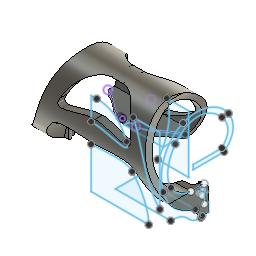
battery (Autodesk Fusion 360 design; units mm, degrees)
Autodesk Fusion 360 part; units mm, degrees
sketch "Skizze5" plane through (0, 0, 0) normal (0, 0, 1) x (1, 0, 0)
  line L0 (28.5, 22, 10) -> (28.5, 20, 10)
  line L1 (28.5, 20, 10) -> (29.5, 21, 10)
  line L2 (29.5, 21, 10) -> (29.5, 19, 10)
  line L3 (28.5, 22, 10) -> (31, 22, 10)
  line L4 (31, 22, 10) -> (31, 19, 10)
  line L5 (29.5, 19, 10) -> (31, 19, 10)
sketch "Skizze6" plane through (0, 0, 0) normal (1, 0, 0) x (0, 1, 0)
  line L0 (29, 22, 31) -> (15, 22, 31)
  line L1 (15, 22, 31) -> (15, 24, 31)
  spline S0 degree 5 poles (14, 14, 31) (13.4292, 14.0943, 31) (12.3218, 14.3255, 31) (10.7626, 14.7996, 31) (8.8887, 15.6876, 31) (6.9008, 17.2273, 31) (5.2976, 19.1966, 31) (4.1324, 21.5861, 31) (3.4909, 24.3735, 31) (3.4767, 27.5066, 31) (4.1857, 30.8831, 31) (5.682, 34.3253, 31) (7.9761, 37.5659, 31) (10.9879, 40.2008, 31) (14.6077, 41.7896, 31) (18.6539, 41.9776, 31) (22.843, 40.5947, 31) (26.7442, 37.7833, 31) (29.7595, 34.0835, 31) (31.0103, 30.6651, 31) (30.6995, 27.8746, 31) (29.6969, 26.1358, 31) (28.8446, 25.0136, 31) (28.2808, 24.3276, 31) (28, 24, 31) knots 0 0 0 0 0 0 0.05 0.1 0.15 0.2 0.25 0.3 0.35 0.4 0.45 0.5 0.55 0.6 0.65 0.7 0.75 0.8 0.85 0.9 0.95 1 1 1 1 1 1
  line L2 (23, 42, 31) -> (33, 30, 31)
  line L3 (31, 27.5, 31) -> (25, 20.5, 31)
  line L4 (15, 24, 31) -> (28, 24, 31)
  line L5 (3.1603, 30.7591, 31) -> (10.8397, 41.2409, 31)
  line L6 (14, 14, 31) -> (20, 14, 31)
  spline S1 degree 5 poles (16, 6.056, 31) (15.2365, 6.3099, 31) (13.7317, 6.851, 31) (11.5407, 7.7632, 31) (8.7707, 9.2347, 31) (5.6767, 11.7695, 31) (3.1232, 15.2227, 31) (1.3063, 19.671, 31) (0.4544, 24.7581, 31) (0.7322, 29.8853, 31) (2.1659, 34.6408, 31) (4.6898, 38.6535, 31) (8.1453, 41.6577, 31) (12.2989, 43.4702, 31) (16.8454, 44.0079, 31) (21.4291, 43.2885, 31) (25.6792, 41.4221, 31) (29.2431, 38.6264, 31) (31.8178, 35.1939, 31) (33.1909, 31.5811, 31) (33.2558, 28.0905, 31) (32.2282, 25.503, 31) (30.8496, 23.6989, 31) (29.6614, 22.5563, 31) (29, 22, 31) knots 0 0 0 0 0 0 0.05 0.1 0.15 0.2 0.25 0.3 0.35 0.4 0.45 0.5 0.55 0.6 0.65 0.7 0.75 0.8 0.85 0.9 0.95 1 1 1 1 1 1
  line L7 (27.7347, 40.9821, 31) -> (34.2653, 31.0179, 31)
  line L8 (20, 6.056, 31) -> (20, 14, 31)
  line L9 (20, 6.056, 31) -> (22, 6.056, 31)
  line L10 (22, 6.056, 31) -> (22, 2, 31)
  line L11 (22, 2, 31) -> (19, 2, 31)
  spline S2 degree 5 poles (16, 6.056, 31) (16.2546, 6.0322, 31) (16.6994, 5.9105, 31) (17.1738, 5.5054, 31) (17.4946, 4.6097, 31) (17.6958, 3.2925, 31) (17.9734, 2.4316, 31) (18.3867, 2.076, 31) (18.7765, 1.9987, 31) (19, 2, 31) knots 0 0 0 0 0 0 0.2 0.4 0.6 0.8 1 1 1 1 1 1
  line L12 (15.4436, 6.108, 31) -> (16.5564, 6.0041, 31)
  line L13 (21.582, 4.2, 31) -> (10.418, 7.912, 31)
  line L14 (18.527, 1.9972, 31) -> (19.473, 2.0028, 31)
  line L15 (3.2202, 13.6342, 31) -> (-0.2202, 26.3658, 31)
  point P0 (5, 20)
  point P1 (7, 36)
  point P2 (28, 36)
  point P3 (1.5, 20)
  point P4 (10.5, 42.5)
  point P5 (31, 36)
extrude "Extrusion7" add sketch "Skizze6" against normal blind 31 contours L0 S0 L3 L6 S1 L8 L9 L10 L11 S2 | L0 L1 L3 L4 in plane through (31, 0, 0) normal (1, 0, 0)
sketch "Skizze12" plane through (0, 0, 0) normal (0, 1, 0) x (1, 0, 0)
  spline S0 degree 5 poles (19, -44) (19.4014, -43.1972) (20.1835, -41.3933) (21.2947, -38.0927) (22.7054, -32.7345) (24.6444, -25.4556) (26.6558, -20.0543) (28.6185, -16.6927) (30.1662, -14.8338) (31, -14) knots 0 0 0 0 0 0 0.2 0.4 0.6 0.8 1 1 1 1 1 1
  line L0 (29, -16) -> (33, -12)
  line L1 (18, -46) -> (20, -42)
  line L2 (19, -44) -> (31, -44)
  line L3 (31, -44) -> (31, -14)
  line L4 (-0.0001, -5.5001) -> (26, -5.5)
  spline S1 degree 5 poles (0, -32.8037) (0.8217, -32.8037) (2.5317, -32.7064) (5.2959, -32.269) (9.2266, -31.2652) (13.7149, -30.1242) (16.0721, -30.121) (16.6063, -31.1017) (16.3108, -32.2798) (16, -33) knots 0 0 0 0 0 0 0.2 0.4 0.6 0.8 1 1 1 1 1 1
  line L5 (16.4469, -31.9643) -> (15.5531, -34.0358)
  line L6 (-2, -32.8037) -> (2, -32.8037)
  spline S2 degree 5 poles (0, -24) (0.3849, -24) (1.3509, -24.0275) (3.3883, -24.1509) (7.043, -24.4207) (12.1145, -24.6156) (15.6276, -24.3209) (17.4643, -23.6442) (18.2499, -22.952) (18.5328, -22.5457) knots 0 0 0 0 0 0 0.2 0.4 0.6 0.8 1 1 1 1 1 1
  line L7 (-1, -24) -> (1, -24)
  line L8 (17.9104, -23.4395) -> (19.1552, -21.6519)
  line L9 (0, -32.8037) -> (0, -43)
  line L10 (2.5307, -43) -> (0, -43)
  line L11 (0, -24) -> (-0.0001, -5.5001)
  spline S3 degree 5 poles (2.5307, -43) (3.6159, -43) (5.6316, -42.8704) (8.1912, -42.2877) (10.8004, -40.8516) (13.1429, -38.4002) (14.5252, -36.2271) (15.346, -34.5996) (15.7979, -33.5306) (16, -33) knots 0 0 0 0 0 0 0.2 0.4 0.6 0.8 1 1 1 1 1 1
  line L12 (-0.9385, -43) -> (6, -43)
  line L13 (15.3419, -34.7276) -> (16.6581, -31.2724)
  spline S4 degree 5 poles (18.5328, -22.5457) (19.0523, -21.9996) (20.0516, -20.8648) (21.4317, -19.0345) (23.0464, -16.3761) (24.6704, -12.8291) (25.5634, -9.9079) (25.9206, -7.7051) (26, -6.2353) (26, -5.5) knots 0 0 0 0 0 0 0.2 0.4 0.6 0.8 1 1 1 1 1 1
  line L14 (17.818, -23.2971) -> (19.2477, -21.7942)
  line L15 (26, -6.5) -> (26, -4.5)
  constraint midpoint S0.end L0
  constraint midpoint S0.start L1
  constraint horizontal L2
  constraint perpendicular L2 L3
  constraint midpoint S1.end L5
  constraint midpoint S1.start L6
  constraint midpoint S2.start L7
  constraint midpoint S2.end L8
  constraint vertical L9
  constraint midpoint L10.start L12
  constraint midpoint S1.end L13
  constraint midpoint S2.end L14
  constraint midpoint L4.end L15
extrude "Extrusion18" cut sketch "Skizze12" along normal blind 41 contours S0 L2 L3
sketch "Skizze13" plane through (0, 15, 0) normal (0, -1, 0) x (1, 0, 0)
  spline S0 degree 5 poles (19.0823, 44) (19.4595, 43.1779) (20.0457, 41.4161) (20.4207, 38.4208) (20.0597, 33.8638) (18.7148, 27.8577) (17.2903, 23.3638) (16.1578, 20.458) (15.3883, 18.7767) (15, 18) knots 0 0 0 0 0 0 0.2 0.4 0.6 0.8 1 1 1 1 1 1
  line L0 (16, 20) -> (14, 16)
  line L1 (18.1646, 46) -> (20, 42)
  line L2 (19.0823, 44) -> (29, 44)
  line L3 (29, 44) -> (29, 18)
  line L4 (29, 18) -> (15, 18)
  constraint midpoint S0.end L0
  constraint midpoint S0.start L1
  constraint horizontal L2
  constraint perpendicular L2 L3
  constraint perpendicular L3 L4
extrude "Extrusion19" cut sketch "Skizze13" against normal blind 26
sketch "Skizze14" plane through (0, 0, 24) normal (0, 0, 1) x (-1, 0, 0)
  spline S0 degree 5 poles (-17.4202, -25) (-16.6728, -24.6912) (-15.252, -24.0265) (-13.3422, -22.8883) (-11.1577, -21.1644) (-8.688, -19.043) (-6.6337, -17.748) (-4.9085, -17.2179) (-3.6536, -17.1) (-3, -17.1) knots 0 0 0 0 0 0 0.2 0.4 0.6 0.8 1 1 1 1 1 1
  line L0 (-5, -17.1) -> (-1, -17.1)
  line L1 (-19.8403, -26) -> (-15, -24)
  line L2 (-17.4202, -25) -> (-17.4202, -15)
  line L3 (-17.4202, -15) -> (0, -15)
  line L4 (0, -15) -> (0, -17.1)
  line L5 (0, -17.1) -> (-3, -17.1)
  constraint midpoint L0 S0.end
  constraint midpoint S0.start L1
  constraint vertical L2
  constraint perpendicular L2 L3
  constraint perpendicular L3 L4
  constraint perpendicular L4 L5
extrude "Extrusion20" cut sketch "Skizze14" against normal blind 2
sketch "Skizze15" plane through (0, 0, 0) normal (0, 0, 1) x (1, 0, 0)
  spline S0 degree 5 poles (29.5, 20) (29.5, 19.2404) (29.3856, 17.9813) (28.8714, 16.8719) (27.6352, 16.6275) (25.7648, 16.9243) (24.5286, 16.3282) (24.0144, 14.7202) (23.9, 13.0127) (23.9, 12) knots 0 0 0 0 0 0 0.2 0.4 0.6 0.8 1 1 1 1 1 1
  line L0 (29.5, 23) -> (29.5, 17)
  line L1 (23.9, 16) -> (23.9, 8)
  line L2 (23.9, 12) -> (-1.0036, 12)
  line L3 (-1.0036, 12) -> (-1.0036, 22)
  line L4 (-1.0036, 22) -> (29.5, 22)
  line L5 (29.5, 22) -> (29.5, 20)
  constraint midpoint S0.start L0
  constraint midpoint S0.end L1
  constraint horizontal L2
  constraint vertical L3
  constraint coincident L0 L4.end
  constraint perpendicular L0 L4
extrude "Extrusion21" cut sketch "Skizze15" along normal blind 14.5
extrude "Extrusion22" cut sketch "Skizze12" along normal blind 14 contours L4 S2 L11 S4 L14 | S2 L14
extrude "Extrusion28" add sketch "Skizze5" along normal blind 4 and the other way blind 4 contours L0 L1 L2 L3 L4 L5 in plane through (0, 0, 10) normal (0, 0, 1)
extrude "Extrusion31" cut sketch "Skizze12" along normal blind 35 contours S1 L9 L10 S3 L12 L13 | S1 L13
fillet "Abrundung1" radius 3 1 edges at (29.75, 22, 14)
mirror "Spiegeln3" about plane through (0, 0, 0) normal (1, 0, 0) of bodies 1 merged
sketch "Skizze18" plane through (0, 0, 0) normal (0, 1, 0) x (1, 0, 0)
  spline S0 degree 5 poles (4, -24, 40) (4.7956, -24.0809, 40) (6.3652, -24.3065, 40) (8.654, -24.8367, 40) (11.5816, -25.9308, 40) (14.7912, -27.8948, 40) (16.9808, -30.2955, 40) (16.7367, -32.7557, 40) (12.2331, -34.6736, 40) (4.4971, -35.7241, 40) (-4.51, -35.7262, 40) (-12.2429, -34.6784, 40) (-16.7411, -32.7596, 40) (-16.9788, -30.2941, 40) (-14.7843, -27.8881, 40) (-11.5729, -25.9218, 40) (-8.6468, -24.8291, 40) (-6.361, -24.3019, 40) (-4.7941, -24.0792, 40) (-4, -24, 40) knots 0 0 0 0 0 0 0.06666667 0.13333333 0.2 0.26666667 0.33333333 0.4 0.46666667 0.53333333 0.6 0.66666667 0.73333333 0.8 0.86666667 0.93333333 1 1 1 1 1 1
  line L0 (4, -24, 40) -> (-4, -24, 40)
  line L1 (16.479, -29.8606, 40) -> (16.521, -32.1394, 40)
  line L2 (-16.5238, -32.1413, 40) -> (-16.4762, -29.8587, 40)
  point P0 (16.5, -31)
  point P1 (-16.5, -31)
extrude "Extrusion29" cut sketch "Skizze18" against normal blind 28 contours S0 L0 in plane through (0, 40, 0) normal (0, 1, 0)
sketch "Skizze19" plane through (0, 0, 24) normal (0, 0, 1) x (-1, 0, 0)
  line L0 (4, -28) -> (17.4202, -28)
  line L1 (17.4202, -25) -> (17.4202, -28)
  line L2 (-17.4202, -25) -> (-17.4202, -28)
  line L3 (-17.4202, -28) -> (-4, -28)
  line L4 (-4, -28) -> (-4, -30.9687)
  line L5 (4, -30.9687) -> (-4, -30.9687)
  line L6 (4, -30.9687) -> (4, -28)
  line L7 (3, -17.1) -> (-3, -17.1)
  spline S0 degree 5 poles (4, -17.1578) (4.4262, -17.2082) (5.444, -17.3985) (6.9556, -17.9537) (8.8431, -19.1761) (11.1577, -21.1644) (13.3422, -22.8883) (15.252, -24.0265) (16.6728, -24.6912) (17.4202, -25) knots -0.937232 -0.937232 -0.937232 -0.937232 -0.937232 -0.937232 -0.8 -0.6 -0.4 -0.2 0 0 0 0 0 0
  spline S1 degree 5 poles (-3, -17.1) (-3.2051, -17.1) (-3.4077, -17.1058) (-3.6077, -17.1174) (-3.8051, -17.1348) (-4, -17.1578) knots -1 -1 -1 -1 -1 -1 -0.937232 -0.937232 -0.937232 -0.937232 -0.937232 -0.937232
  spline S2 degree 5 poles (3, -17.1) (3.2051, -17.1) (3.4077, -17.1058) (3.6077, -17.1174) (3.8051, -17.1348) (4, -17.1578) knots -1 -1 -1 -1 -1 -1 -0.937232 -0.937232 -0.937232 -0.937232 -0.937232 -0.937232
  spline S3 degree 5 poles (-4, -17.1578) (-4.4262, -17.2082) (-5.444, -17.3985) (-6.9556, -17.9537) (-8.8431, -19.1761) (-11.1577, -21.1644) (-13.3422, -22.8883) (-15.252, -24.0265) (-16.6728, -24.6912) (-17.4202, -25) knots -0.937232 -0.937232 -0.937232 -0.937232 -0.937232 -0.937232 -0.8 -0.6 -0.4 -0.2 0 0 0 0 0 0
